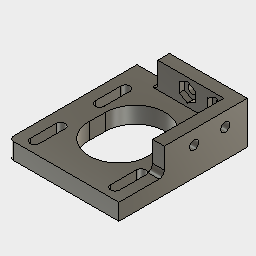
bart pro xl y motor mount v3 (Autodesk Fusion 360 design; units mm, degrees)
Autodesk Fusion 360 part; units mm, degrees
sketch "Sketch1" plane through (0, 0, 0) normal (0, 0, 1) x (1, 0, 0)
  line L0 (0, 0) -> (42.5, 0)
  line L1 (42.5, 0) -> (42.5, 49.5)
  line L2 (42.5, 49.5) -> (0, 49.5)
  line L3 (0, 49.5) -> (0, 0)
  line L4 (42.5, 49.5) -> (0, 0) construction
  line L5 (0, 49.5) -> (42.5, 0) construction
  arc A0 (17.357, 20.2158) -> (17.4515, 20.1909) centre (20.3375, 31.3229) ccw
  line L6 (21.25, 49.5) -> (21.25, 38) construction
  line L7 (21.25, 38) -> (21.25, 8.6498) construction
  arc A1 (9.7527, 21.4972) -> (32.6042, 19.4227) centre (21.25, 21.248) ccw
  line L8 (32.6042, 29.9934) -> (32.6042, 20)
  arc A2 (32.6042, 29.9934) -> (9.8814, 27.434) centre (21.3813, 27.4842) ccw
  line L9 (32.6042, 20) -> (32.6042, 19.4227)
  line L10 (9.8944, 28.0329) -> (9.7527, 21.4972)
  line L11 (42.5, 48.2146) -> (36.78, 48.2146) construction
  line L12 (36.78, 48.2146) -> (36.78, 46)
  line L13 (36.78, 46) -> (36.78, -1) construction
  line L14 (36.78, -1) -> (5.78, -1) construction
  line L15 (5.78, -1) -> (5.78, 51) construction
  line L16 (21.25, 24.75) -> (21.25, 40.25)
  line L17 (21.25, 34.2561) -> (4, 34.2561) construction
  line L18 (21.25, 24.75) -> (-10, 24.75) construction
  line L19 (-10, 24.75) -> (-10, 9.25) construction
  line L20 (-10, 9.25) -> (46, 9.25) construction
  line L21 (35.03, 14.25) -> (35.03, 4.25)
  arc A3 (35.03, 4.25) -> (38.53, 4.25) centre (36.78, 4.25) ccw
  line L22 (38.53, 4.25) -> (38.53, 14.25)
  arc A4 (38.53, 14.25) -> (35.03, 14.25) centre (36.78, 14.25) ccw
  line L23 (36.78, 14.25) -> (36.78, 4.25) construction
  line L24 (7.53, 29.2561) -> (7.53, 39.2561)
  arc A5 (7.53, 39.2561) -> (4.03, 39.2561) centre (5.78, 39.2561) ccw
  line L25 (4.03, 39.2561) -> (4.03, 29.2561)
  arc A6 (4.03, 29.2561) -> (7.53, 29.2561) centre (5.78, 29.2561) ccw
  line L26 (5.78, 29.2561) -> (5.78, 39.2561) construction
  line L27 (7.53, 4.25) -> (7.53, 14.25)
  arc A7 (7.53, 14.25) -> (4.03, 14.25) centre (5.78, 14.25) ccw
  line L28 (4.03, 14.25) -> (4.03, 4.25)
  arc A8 (4.03, 4.25) -> (7.53, 4.25) centre (5.78, 4.25) ccw
  line L29 (5.78, 4.25) -> (5.78, 14.25) construction
  dimension "d1" = 42.5
  dimension "d2" = 49.5
  dimension "d8" = 5.72
  dimension "d10" = 3.5
  dimension "d11" = 3.5
  dimension "d12" = 3.5
  constraint horizontal L0
  constraint vertical L1
  constraint horizontal L2
  constraint vertical L3
  constraint midpoint L2
  constraint vertical L7
  constraint vertical L8
  constraint parallel L8 L9
  constraint coincident A2
  constraint tangent A1 L10
  constraint coincident L10
  constraint coincident L1
  constraint perpendicular L11 L12
  constraint perpendicular L0 L13
  constraint perpendicular L2 L15
  constraint midpoint L5
  constraint coincident L16
  constraint coincident L7
  constraint perpendicular L3 L17
  constraint perpendicular L16 L18
  constraint perpendicular L1 L20
  constraint tangent L21 A3
  constraint tangent A3 L22
  constraint parallel L21 L22
  constraint tangent L22 A4
  constraint tangent L21 A4
  constraint midpoint L23
  constraint tangent L24 A5
  constraint tangent A5 L25
  constraint parallel L24 L25
  constraint tangent L25 A6
  constraint tangent L24 A6
  constraint midpoint L26
  constraint tangent L27 A7
  constraint tangent A7 L28
  constraint parallel L27 L28
  constraint tangent L28 A8
  constraint tangent L27 A8
  constraint midpoint L29
  measures "d10" diameter of A3
  measures "d11" diameter of A5
  measures "d12" diameter of A7
extrude "Extrude1" add sketch "Sketch1" along normal blind 6.35
sketch "Sketch2" plane through (0, 0, 6.35) normal (0, 0, 1) x (-1, 0, 0)
  arc A0 (-4.03, -29.2561) -> (-7.53, -29.2561) centre (-5.78, -29.2561) ccw
  line L0 (-4.03, -29.2561) -> (-4.03, -39.2561)
  arc A1 (-7.53, -39.2561) -> (-4.03, -39.2561) centre (-5.78, -39.2561) ccw
  line L1 (-7.53, -39.2561) -> (-7.53, -29.2561)
  arc A2 (-38.53, -14.25) -> (-35.03, -14.25) centre (-36.78, -14.25) ccw
  line L2 (-38.53, -14.25) -> (-38.53, -4.25)
  arc A3 (-35.03, -4.25) -> (-38.53, -4.25) centre (-36.78, -4.25) ccw
  line L3 (-35.03, -4.25) -> (-35.03, -14.25)
  arc A4 (-32.6042, -29.9934) -> (-9.8814, -27.434) centre (-21.3813, -27.4842) ccw
  line L4 (-32.6042, -29.9934) -> (-32.6042, -19.4227)
  arc A5 (-9.7527, -21.4972) -> (-32.6042, -19.4227) centre (-21.25, -21.248) ccw
  line L5 (-9.7527, -21.4972) -> (-9.8814, -27.434)
  arc A6 (-4.03, -4.25) -> (-7.53, -4.25) centre (-5.78, -4.25) ccw
  line L6 (-4.03, -4.25) -> (-4.03, -14.25)
  arc A7 (-7.53, -14.25) -> (-4.03, -14.25) centre (-5.78, -14.25) ccw
  line L7 (-7.53, -14.25) -> (-7.53, -4.25)
  line L8 (0, -49.5) -> (0, 0)
  line L9 (0, 0) -> (-42.5, 0)
  line L10 (-42.5, 0) -> (-42.5, -49.5)
  line L11 (-42.5, -49.5) -> (0, -49.5)
  line L12 (-42.5, -49.5) -> (-38, -49.5)
  line L13 (-38, -45) -> (-38, -17.5)
  line L14 (-38, -17.5) -> (-42.5, -17.5)
  line L15 (-42.5, -17.5) -> (-42.5, -49.5)
  line L16 (-42.5, -49.5) -> (-12.5, -49.5)
  line L17 (-12.5, -49.5) -> (-12.5, -45)
  line L18 (-12.5, -45) -> (-38, -45)
  line L19 (-42.5, -45) -> (-42.5, -49.5)
  dimension "d15" = 32
  dimension "d16" = 4.5
  dimension "d17" = 30
  constraint horizontal L12
  constraint vertical L13
  constraint horizontal L14
  constraint vertical L15
  constraint horizontal L16
  constraint vertical L17
  constraint horizontal L18
  constraint vertical L19
extrude "Extrude2" add sketch "Sketch2" along normal blind 10 contours L10 L11 L12 L13 L14 L15 L16 L17 L18 L19
sketch "Sketch3" plane through (42.5, 0, 0) normal (1, 0, 0) x (0, 1, 0)
  line L0 (0, 0) -> (49.5, 0)
  line L1 (49.5, 0) -> (49.5, 16.35)
  line L2 (49.5, 16.35) -> (17.5, 16.35)
  line L3 (17.5, 16.35) -> (17.5, 6.35)
  line L4 (17.5, 6.35) -> (0, 6.35)
  line L5 (0, 6.35) -> (0, 0)
  line L6 (55, 16) -> (55, 11) construction
  line L7 (55, 11) -> (53, 11)
  line L8 (53, 11) -> (8, 11) construction
  line L9 (49.5, 8.175) -> (41, 8.175) construction
  line L10 (41, 8.175) -> (41, 13) construction
  line L11 (41, 13) -> (29, 13) construction
  line L12 (29, 13) -> (29, 7) construction
  dimension "d20" = 5
  constraint perpendicular L6 L7
  constraint perpendicular L6 L8
  constraint midpoint L1
  constraint perpendicular L8 L10
  constraint perpendicular L8 L12
  constraint coincident L10
  constraint coincident L8
  constraint coincident L12
hole "Hole1" at (42.5, 41, 11) direction (-1, 0, 0) diameter 3.5 end through all
hole "Hole2" at (42.5, 29, 11) direction (-1, 0, 0) diameter 3.5 end through all
sketch "Sketch4" plane through (38, 0, 0) normal (-1, 0, 0) x (0, -1, 0)
  circle A0 centre (-29, 11) radius 1.75
  circle A1 centre (-41, 11) radius 1.75
  line L0 (-45, 6.35) -> (-17.5, 6.35)
  line L1 (-17.5, 6.35) -> (-17.5, 16.35)
  line L2 (-17.5, 16.35) -> (-45, 16.35)
  line L3 (-45, 16.35) -> (-45, 6.35)
  line L4 (-44.15, 9.1813) -> (-41, 7.3627)
  line L5 (-41, 7.3627) -> (-37.85, 9.1813)
  line L6 (-37.85, 9.1813) -> (-37.85, 12.8187)
  line L7 (-37.85, 12.8187) -> (-41, 14.6373)
  line L8 (-41, 14.6373) -> (-44.15, 12.8187)
  line L9 (-44.15, 12.8187) -> (-44.15, 9.1813)
sketch "Sketch5" plane through (38, 0, 0) normal (-1, 0, 0) x (0, -1, 0)
  circle A0 centre (-29, 11) radius 1.75
  line L0 (-45, 6.35) -> (-17.5, 6.35)
  line L1 (-17.5, 6.35) -> (-17.5, 16.35)
  line L2 (-17.5, 16.35) -> (-45, 16.35)
  line L3 (-45, 16.35) -> (-45, 6.35)
  line L4 (-32.15, 9.1813) -> (-29, 7.3627)
  line L5 (-29, 7.3627) -> (-25.85, 9.1813)
  line L6 (-25.85, 9.1813) -> (-25.85, 12.8187)
  line L7 (-25.85, 12.8187) -> (-29, 14.6373)
  line L8 (-29, 14.6373) -> (-32.15, 12.8187)
  line L9 (-32.15, 12.8187) -> (-32.15, 9.1813)
  circle A1 centre (-41, 11) radius 1.75
sketch "Sketch6" plane through (0, 49.5, 0) normal (0, 1, 0) x (-1, 0, 0)
  line L0 (-42.5, 0) -> (0, 0)
  line L1 (0, 0) -> (0, 6.35)
  line L2 (0, 6.35) -> (-12.5, 6.35)
  line L3 (-12.5, 6.35) -> (-12.5, 16.35)
  line L4 (-12.5, 16.35) -> (-42.5, 16.35)
  line L5 (-42.5, 16.35) -> (-42.5, 0)
  line L6 (-38, 16.35) -> (-42.5, 16.35)
  line L7 (-40.25, 16.35) -> (-40.25, 11.35) construction
  line L8 (-40.25, 11.35) -> (-4, 11.35) construction
  line L9 (-42.5, 8.175) -> (-34.7, 8.175) construction
  line L10 (-34.7, 8.175) -> (-34.7, 13) construction
  line L11 (-34.7, 13) -> (-23.9, 13) construction
  line L12 (0, 6.35) -> (-42.5, 6.35)
  line L13 (-23.9, 13) -> (-23.9, 6.35) construction
  constraint midpoint L6
  constraint perpendicular L3 L8
  constraint midpoint L5
  constraint perpendicular L8 L10
  constraint coincident L12
  constraint perpendicular L8 L13
  constraint coincident L13
  constraint coincident L8
  constraint coincident L10
hole "Hole3" at (23.9, 49.5, 11.35) direction (0, -1, 0) diameter 3.5 end through all
hole "Hole4" at (34.7, 49.5, 11.35) direction (0, -1, 0) diameter 3.5 end through all
sketch "Sketch7" plane through (0, 45, 0) normal (0, -1, 0) x (1, 0, 0)
  circle A0 centre (34.7, 11.35) radius 1.75
  circle A1 centre (23.9, 11.35) radius 1.75
  line L0 (12.5, 6.35) -> (38, 6.35)
  line L1 (38, 6.35) -> (38, 16.35)
  line L2 (38, 16.35) -> (12.5, 16.35)
  line L3 (12.5, 16.35) -> (12.5, 6.35)
  line L4 (37.86, 13.1513) -> (34.72, 14.9873)
  line L5 (34.72, 14.9873) -> (31.5601, 13.186)
  line L6 (31.5601, 13.186) -> (31.54, 9.5487)
  line L7 (31.54, 9.5487) -> (34.68, 7.7127)
  line L8 (34.68, 7.7127) -> (37.8399, 9.514)
  line L9 (37.8399, 9.514) -> (37.86, 13.1513)
extrude "Extrude5" cut sketch "Sketch7" against normal blind 2 contours L4 L5 L6 L7 L8 L9
sketch "Sketch8" plane through (0, 45, 0) normal (0, -1, 0) x (1, 0, 0)
  line L0 (34.72, 14.9873) -> (37.86, 13.1513)
  line L1 (37.86, 13.1513) -> (37.8399, 9.514)
  line L2 (37.8399, 9.514) -> (34.68, 7.7127)
  line L3 (34.68, 7.7127) -> (31.54, 9.5487)
  line L4 (31.54, 9.5487) -> (31.5601, 13.186)
  line L5 (31.5601, 13.186) -> (34.72, 14.9873)
  circle A0 centre (23.9, 11.35) radius 1.75
  line L6 (12.5, 6.35) -> (38, 6.35)
  line L7 (38, 6.35) -> (38, 16.35)
  line L8 (38, 16.35) -> (12.5, 16.35)
  line L9 (12.5, 16.35) -> (12.5, 6.35)
  line L10 (20.75, 9.5313) -> (23.9, 7.7127)
  line L11 (23.9, 7.7127) -> (27.05, 9.5313)
  line L12 (27.05, 9.5313) -> (27.05, 13.1687)
  line L13 (27.05, 13.1687) -> (23.9, 14.9873)
  line L14 (23.9, 14.9873) -> (20.75, 13.1687)
  line L15 (20.75, 13.1687) -> (20.75, 9.5313)
extrude "Extrude6" cut sketch "Sketch8" against normal blind 2 contours L10 L11 L12 L13 L14 L15
fillet "Fillet1" radius 2 1 edges at (0, 0, 3.175)
extrude "Extrude7" cut sketch "Sketch5" against normal blind 2 contours L4 L5 L6 L7 L8 L9
extrude "Extrude8" cut sketch "Sketch4" against normal blind 2 contours L4 L5 L6 L7 L8 L9
fillet "Fillet2" radius 2 1 edges at (12.5, 47.25, 6.35)
fillet "Fillet3" radius 2 1 edges at (40.25, 17.5, 6.35)
